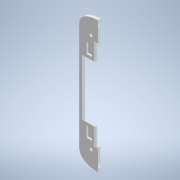
# Autodesk Inventor part: back_diffuser
Saved by Autodesk Inventor 2022 (Build 260153000, 153)
## iProperties
Created: 2024-12-22
Part Number: back_diffuser
Material: Типовые
Document SubType Name: Modeling
Designer: Andrey
Density: 1 g/cm^3
Appearance: По умолчанию
Author: Andrey
Autodesk Inventor part; units mm, degrees
ref_plane "YZ Plane" through (0, 0, 0) normal (1, 0, 0) x (0, 1, 0)
ref_plane "XZ Plane" through (0, 0, 0) normal (0, 1, 0) x (-1, 0, 0)
ref_plane "XY Plane" through (0, 0, 0) normal (0, 0, 1) x (1, 0, 0)
sketch "Эскиз1" plane through (0, 0, 0) normal (0, 0, 1) x (1, 0, 0)
  arc A0 (21.9698, 25.0872) -> (24.9698, 22.0872) centre (24.9698, 25.0872) ccw
  line L0 (24.9698, 22.0872) -> (32.4715, 22.0872)
  arc A1 (35.4715, 19.0872) -> (32.4715, 22.0872) centre (32.4715, 19.0872) ccw
  line L1 (35.4715, 19.0872) -> (35.4715, -12.1128)
  arc A2 (32.4715, -15.1128) -> (35.4715, -12.1128) centre (32.4715, -12.1128) ccw
  line L2 (32.4715, -15.1128) -> (24.9698, -15.1128)
  arc A3 (24.9698, -15.1128) -> (21.9698, -18.1128) centre (24.9698, -18.1128) ccw
  line L3 (21.9698, -18.1128) -> (21.9698, -28.1128)
  line L4 (21.9698, -28.1128) -> (36.9698, -28.1128)
  line L5 (36.9698, -28.1128) -> (36.9698, -40.6128)
  line L6 (36.9698, -40.6128) -> (21.9698, -40.6128)
  line L7 (21.9698, -40.6128) -> (21.9698, -43.5128)
  line L8 (21.9698, -43.5128) -> (58.0248, -43.5128)
  arc A4 (60.0248, -45.5128) -> (58.0248, -43.5128) centre (58.0248, -45.5128) ccw
  line L9 (60.0248, -45.5128) -> (60.0248, -60.8075)
  arc A5 (58.0248, -62.8075) -> (60.0248, -60.8075) centre (58.0248, -60.8075) ccw
  line L10 (58.0248, -62.8075) -> (-57.9752, -62.8075)
  arc A6 (-59.9752, -60.8075) -> (-57.9752, -62.8075) centre (-57.9752, -60.8075) ccw
  line L11 (-59.9752, -60.8075) -> (-59.9752, -45.5128)
  arc A7 (-57.9752, -43.5128) -> (-59.9752, -45.5128) centre (-57.9752, -45.5128) ccw
  line L12 (-57.9752, -43.5128) -> (-22.0457, -43.5128)
  line L13 (-22.0457, -43.5128) -> (-22.0457, -40.6128)
  line L14 (-22.0457, -40.6128) -> (-39.5957, -40.6128)
  line L15 (-39.5957, -40.6128) -> (-39.5957, -29.6128)
  line L16 (-39.5957, -29.6128) -> (-22.0457, -29.6128)
  line L17 (-22.0457, -29.6128) -> (-22.0457, -27.6266)
  line L18 (-22.0457, -27.6266) -> (-23.1715, -27.6266)
  line L19 (-23.1715, -27.6266) -> (-23.1715, -10.2508)
  line L20 (-23.1715, -10.2508) -> (-22.0457, -10.2508)
  line L21 (-22.0457, -10.2508) -> (-22.0457, -5.0128)
  line L22 (-22.0457, -5.0128) -> (-25.0457, -5.0128)
  line L23 (-25.0457, -5.0128) -> (-25.0457, 4.9872)
  line L24 (-25.0457, 4.9872) -> (-22.0457, 4.9872)
  line L25 (-22.0457, 4.9872) -> (-22.0457, 10.2252)
  line L26 (-22.0457, 10.2252) -> (-23.1715, 10.2252)
  line L27 (-23.1715, 10.2252) -> (-23.1715, 27.601)
  line L28 (-23.1715, 27.601) -> (-22.0457, 27.601)
  line L29 (-22.0457, 27.601) -> (-22.0457, 43.4872)
  line L30 (-22.0457, 43.4872) -> (-57.9752, 43.4872)
  arc A8 (-59.9752, 45.4872) -> (-57.9752, 43.4872) centre (-57.9752, 45.4872) ccw
  line L31 (-59.9752, 45.4872) -> (-59.9752, 60.782)
  arc A9 (-57.9752, 62.782) -> (-59.9752, 60.782) centre (-57.9752, 60.782) ccw
  line L32 (-57.9752, 62.782) -> (58.0248, 62.782)
  arc A10 (60.0248, 60.782) -> (58.0248, 62.782) centre (58.0248, 60.782) ccw
  line L33 (60.0248, 60.782) -> (60.0248, 45.4872)
  arc A11 (58.0248, 43.4872) -> (60.0248, 45.4872) centre (58.0248, 45.4872) ccw
  line L34 (58.0248, 43.4872) -> (21.9698, 43.4872)
  line L35 (21.9698, 43.4872) -> (21.9698, 25.0872)
  circle A12 centre (-51.6466, 22.9919) radius 1.5
  circle A13 centre (-51.6466, -23.0174) radius 1.5
  line L36 (-50.445, -3.8128) -> (-50.445, 15.6872)
  arc A14 (-47.445, 18.6872) -> (-50.445, 15.6872) centre (-47.445, 15.6872) ccw
  line L37 (-47.445, 18.6872) -> (-33.6813, 18.6872)
  arc A15 (-30.6813, 15.6872) -> (-33.6813, 18.6872) centre (-33.6813, 15.6872) ccw
  line L38 (-30.6813, 15.6872) -> (-30.6813, -3.8128)
  arc A16 (-33.6813, -6.8128) -> (-30.6813, -3.8128) centre (-33.6813, -3.8128) ccw
  line L39 (-33.6813, -6.8128) -> (-47.445, -6.8128)
  arc A17 (-50.445, -3.8128) -> (-47.445, -6.8128) centre (-47.445, -3.8128) ccw
  line L40 (60.4248, -29.3128) -> (60.4248, -21.9128)
  line L41 (60.4248, -21.9128) -> (74.9248, -21.9128)
  line L42 (74.9248, -21.9128) -> (74.9248, -29.3128)
  line L43 (74.9248, -29.3128) -> (60.4248, -29.3128)
  line L44 (60.4248, 21.8872) -> (60.4248, 29.2872)
  line L45 (60.4248, 29.2872) -> (74.9248, 29.2872)
  line L46 (74.9248, 29.2872) -> (74.9248, 21.8872)
  line L47 (74.9248, 21.8872) -> (60.4248, 21.8872)
  line L48 (79.0248, -17.5128) -> (68.0248, -17.5128)
  line L49 (68.0248, -17.5128) -> (68.0248, -6.0128)
  line L50 (68.0248, -6.0128) -> (63.1715, -6.0128)
  arc A18 (62.1715, -5.0128) -> (63.1715, -6.0128) centre (63.1715, -5.0128) ccw
  line L51 (62.1715, -5.0128) -> (62.1715, 4.9872)
  arc A19 (63.1715, 5.9872) -> (62.1715, 4.9872) centre (63.1715, 4.9872) ccw
  line L52 (63.1715, 5.9872) -> (68.0248, 5.9872)
  line L53 (68.0248, 5.9872) -> (68.0248, 17.4872)
  line L54 (68.0248, 17.4872) -> (79.0248, 17.4872)
  line L55 (79.0248, 17.4872) -> (79.0248, 52.7508)
  spline S0 degree 4 poles (79.0248, 52.7508) (79.0248, 55.4389) (78.6593, 58.1507) (77.2994, 60.4709) (75.0248, 62.2967) knots 0 0 0 0 0 1 1 1 1 1
  spline S1 degree 4 poles (75.0248, 62.2967) (71.8239, 64.8662) (66.8118, 66.4567) (60.2111, 66.782) (55.0248, 66.782) knots 0.415412 0.415412 0.415412 0.415412 0.415412 1 1 1 1 1
  line L56 (-54.9752, 66.782) -> (55.0248, 66.782)
  spline S2 degree 4 poles (-54.9752, 66.782) (-60.1615, 66.782) (-66.7622, 66.4567) (-71.7743, 64.8662) (-74.9752, 62.2967) knots 0 0 0 0 0 0.584588 0.584588 0.584588 0.584588 0.584588
  spline S3 degree 4 poles (-74.9752, 62.2967) (-77.2498, 60.4709) (-78.6098, 58.1507) (-78.9752, 55.4389) (-78.9752, 52.7508) knots 0 0 0 0 0 1 1 1 1 1
  line L57 (-78.9752, 52.7508) -> (-78.9752, -52.7764)
  spline S4 degree 4 poles (-78.9752, -52.7764) (-78.9752, -55.4644) (-78.6098, -58.1763) (-77.2498, -60.4964) (-74.9752, -62.3223) knots 0 0 0 0 0 1 1 1 1 1
  spline S5 degree 4 poles (-74.9752, -62.3223) (-71.7743, -64.8917) (-66.7622, -66.4822) (-60.1615, -66.8075) (-54.9752, -66.8075) knots 0.415412 0.415412 0.415412 0.415412 0.415412 1 1 1 1 1
  line L58 (55.0248, -66.8075) -> (-54.9752, -66.8075)
  spline S6 degree 4 poles (55.0248, -66.8075) (60.2111, -66.8075) (66.8118, -66.4822) (71.8239, -64.8917) (75.0248, -62.3223) knots 0 0 0 0 0 0.584588 0.584588 0.584588 0.584588 0.584588
  spline S7 degree 4 poles (75.0248, -62.3223) (77.2994, -60.4964) (78.6593, -58.1763) (79.0248, -55.4644) (79.0248, -52.7764) knots 0 0 0 0 0 1 1 1 1 1
  line L59 (79.0248, -52.7764) -> (79.0248, -17.5128)
  circle A20 centre (-29.4752, -25.5128) radius 1.25
  circle A21 centre (29.5248, 25.4872) radius 1.25
  circle A22 centre (29.5248, -25.5128) radius 1.25
  circle A23 centre (-29.4752, 25.4872) radius 1.25
  circle A24 centre (-51.6466, 22.9919) radius 2.1
  circle A25 centre (-51.6466, -23.0174) radius 2.1
  line L60 (-72.9752, -28.1266) -> (-39.8957, -28.1266)
  line L61 (-39.8957, 28.101) -> (-72.9752, 28.101)
  line L62 (-39.8957, 28.101) -> (-39.8957, 16.9648)
  ellipse E0 centre (-48.5541, 13.1872) end of major axis (-34.5198, 13.1872) minor radius 4.8 (-39.8957, 16.9648) -> (-62.5883, 13.1872) ccw
  line L63 (-62.5883, 13.1872) -> (-62.5883, -1.3128)
  ellipse E1 centre (-48.5541, -1.3128) end of major axis (-62.5883, -1.3128) minor radius 4.8 (-62.5883, -1.3128) -> (-39.8957, -5.0904) ccw
  line L64 (-39.8957, -5.0904) -> (-39.8957, -28.1266)
  line L65 (-59.9752, -66.667) -> (-59.9752, 66.6415)
  line L66 (-75.9752, -52.7764) -> (-75.9752, 52.7508)
  line L67 (-54.9752, 63.782) -> (55.0248, 63.782)
  line L68 (76.0248, 52.7508) -> (76.0248, 20.4872)
  line L69 (76.0248, 20.4872) -> (65.0248, 20.4872)
  line L70 (65.0248, 20.4872) -> (65.0248, 8.9872)
  line L71 (65.0248, 8.9872) -> (63.1715, 8.9872)
  arc A26 (63.1715, 8.9872) -> (59.1715, 4.9872) centre (63.1715, 4.9872) ccw
  line L72 (59.1715, 4.9872) -> (59.1715, -5.0128)
  arc A27 (59.1715, -5.0128) -> (63.1715, -9.0128) centre (63.1715, -5.0128) ccw
  line L73 (63.1715, -9.0128) -> (65.0248, -9.0128)
  line L74 (65.0248, -9.0128) -> (65.0248, -20.5128)
  line L75 (65.0248, -20.5128) -> (76.0248, -20.5128)
  line L76 (76.0248, -20.5128) -> (76.0248, -52.7764)
  line L77 (55.0248, -63.8075) -> (-54.9752, -63.8075)
  line L78 (-72.9752, -28.1266) -> (-72.9752, 28.101)
  spline S8 degree 5 poles (-73.0972, -59.9828) (-73.6957, -59.5017) (-74.2433, -58.9582) (-74.7152, -58.3353) (-75.4815, -56.9001) (-75.8411, -55.3112) (-75.9357, -54.4671) (-75.9756, -53.6221) (-75.9752, -52.7764) knots 0 0 0 0 0 0 0.475904 0.475904 0.475904 1 1 1 1 1 1
  spline S9 degree 5 poles (-75.9752, 52.7508) (-75.9756, 53.5966) (-75.9357, 54.4415) (-75.8411, 55.2856) (-75.4815, 56.8745) (-74.7152, 58.3097) (-74.2433, 58.9326) (-73.6957, 59.4761) (-73.0972, 59.9572) knots 0 0 0 0 0 0 0.524096 0.524096 0.524096 1 1 1 1 1 1
  spline S10 degree 5 poles (-73.0972, 59.9572) (-71.8214, 60.9817) (-70.3144, 61.7034) (-68.7678, 62.2382) (-65.1123, 63.1767) (-61.3615, 63.5924) (-59.2342, 63.7293) (-57.1048, 63.7818) (-54.9752, 63.782) knots 0 0 0 0 0 0 0.434284 0.434284 0.434284 1 1 1 1 1 1
  spline S11 degree 5 poles (55.0248, 63.782) (57.1544, 63.7818) (59.2838, 63.7293) (61.4111, 63.5924) (65.1619, 63.1767) (68.8174, 62.2382) (70.364, 61.7034) (71.871, 60.9817) (73.1468, 59.9572) knots 0 0 0 0 0 0 0.565716 0.565716 0.565716 1 1 1 1 1 1
  spline S12 degree 5 poles (73.1468, 59.9572) (73.7453, 59.4761) (74.2929, 58.9326) (74.7647, 58.3097) (75.531, 56.8745) (75.8907, 55.2856) (75.9853, 54.4415) (76.0252, 53.5966) (76.0248, 52.7508) knots 0 0 0 0 0 0 0.475904 0.475904 0.475904 1 1 1 1 1 1
  spline S13 degree 5 poles (76.0248, -52.7764) (76.0252, -53.6221) (75.9853, -54.4671) (75.8907, -55.3112) (75.531, -56.9001) (74.7647, -58.3353) (74.2929, -58.9582) (73.7453, -59.5017) (73.1468, -59.9828) knots 0 0 0 0 0 0 0.524096 0.524096 0.524096 1 1 1 1 1 1
  spline S14 degree 5 poles (73.1468, -59.9828) (71.871, -61.0073) (70.364, -61.7289) (68.8174, -62.2638) (65.1619, -63.2022) (61.4111, -63.618) (59.2838, -63.7549) (57.1544, -63.8074) (55.0248, -63.8075) knots 0 0 0 0 0 0 0.434284 0.434284 0.434284 1 1 1 1 1 1
  spline S15 degree 5 poles (-54.9752, -63.8075) (-57.1048, -63.8074) (-59.2342, -63.7549) (-61.3615, -63.618) (-65.1123, -63.2022) (-68.7678, -62.2638) (-70.3144, -61.7289) (-71.8214, -61.0073) (-73.0972, -59.9828) knots 0 0 0 0 0 0 0.565716 0.565716 0.565716 1 1 1 1 1 1
  point P0 (0, 0)
  point P1 (-78.9752, -28.1266)
  point P2 (-78.9752, 28.101)
  point P3 (-59.9752, -63.6611)
  point P4 (-59.9752, 63.6356)
  dimension "d0" = 3
  constraints: 26 end point, 8 parallel, 4 point on circle, 2 centre point, 1 collinear, 38 other
extrude "Выдавливание1" add sketch "Эскиз1" along normal blind 3 contours S10 S9 L66 S8 S15 L65 S5 S4 L57 S3 S2
sketch "Эскиз3" plane through (0, 0, 3) normal (0, 0, 1) x (1, 0, 0)
  line L0 (-78.9752, 52.7508) -> (-78.9752, -52.7764) projected
  line L1 (-59.9752, -66.667) -> (-59.9752, -63.6611) projected
  spline S0 degree 5 poles (-59.9752, -63.6611) (-61.1018, -63.5885) (-62.2267, -63.4897) (-63.3488, -63.36) (-66.084, -62.9528) (-68.7678, -62.2638) (-70.3144, -61.7289) (-71.8214, -61.0073) (-73.0972, -59.9828) knots 0 0 0 0 0 0 0.408481 0.408481 0.408481 1 1 1 1 1 1 projected
  spline S1 degree 5 poles (-73.0972, -59.9828) (-73.6957, -59.5017) (-74.2433, -58.9582) (-74.7152, -58.3353) (-75.4815, -56.9001) (-75.8411, -55.3112) (-75.9357, -54.4671) (-75.9756, -53.6221) (-75.9752, -52.7764) knots 0 0 0 0 0 0 0.475904 0.475904 0.475904 1 1 1 1 1 1 projected
  line L2 (-75.9752, -52.7764) -> (-75.9752, 52.7508) projected
  spline S2 degree 5 poles (-75.9752, 52.7508) (-75.9756, 53.5966) (-75.9357, 54.4415) (-75.8411, 55.2856) (-75.4815, 56.8745) (-74.7152, 58.3097) (-74.2433, 58.9326) (-73.6957, 59.4761) (-73.0972, 59.9572) knots 0 0 0 0 0 0 0.524096 0.524096 0.524096 1 1 1 1 1 1 projected
  spline S3 degree 5 poles (-73.0972, 59.9572) (-71.8214, 60.9817) (-70.3144, 61.7034) (-68.7678, 62.2382) (-66.084, 62.9272) (-63.3488, 63.3345) (-62.2267, 63.4641) (-61.1018, 63.5629) (-59.9752, 63.6355) knots 0 0 0 0 0 0 0.591519 0.591519 0.591519 1 1 1 1 1 1 projected
  line L3 (-59.9752, 63.6356) -> (-59.9752, 66.6415) projected
  line L4 (-39.8957, 28.101) -> (-59.6752, 28.101) projected
  line L5 (-39.8957, 28.101) -> (-39.8957, 16.9648) projected
  circle A0 centre (-51.6466, 22.9919) radius 2.1 projected
  line L6 (-78.9752, -28.1266) -> (-76.3894, -28.1266) projected
  line L7 (-78.9752, 28.101) -> (-78.9752, -28.1266) projected
  line L8 (-76.3894, 28.101) -> (-78.9752, 28.101) projected
  line L9 (-59.9752, -66.667) -> (-59.9752, -63.6611) projected
  line L10 (-59.9752, -63.6611) -> (-59.9752, 63.6356)
  line L11 (-59.9752, -28.4266) -> (-78.9752, -28.4266)
  line L12 (-59.9752, 28.401) -> (-78.9752, 28.401)
  line L13 (-76.3894, -28.1266) -> (-76.3894, 28.101) projected
  ellipse E0 centre (-48.5541, 13.1872) end of major axis (-34.5198, 13.1872) minor radius 4.8 (-39.8957, 16.9648) -> (-59.6752, 16.115) ccw projected
  line L14 (-59.6752, 16.115) -> (-59.6752, 28.101) projected
  point P0 (0, 0)
  point P1 (-75.9752, 28.401)
  point P2 (-75.9752, -28.4266)
  dimension "d5" = 0.3
  constraints: 6 end point, 4 point on line, 2 perpendicular, 1 collinear, 9 other
  measures "d5" distance between parallel lines of L12 L4
extrude "Выдавливание3" add sketch "Эскиз3" against normal blind 0.4 contours L2 S2 S3 L10 L12 | L11 L10 S0 S1 L2
sketch "Эскиз4" plane through (0, 0, 2.6) normal (0, 0, -1) x (-1, 0, 0)
  circle A0 centre (66.9752, -50.0128) radius 1.35
  circle A1 centre (66.9752, 49.9872) radius 1.35
  arc A2 (57.945, -33.5297) -> (52.945, -33.5297) centre (55.445, -33.5297) ccw
  line L0 (57.945, -33.5297) -> (57.945, -38.6097)
  arc A3 (52.945, -38.6097) -> (57.945, -38.6097) centre (55.445, -38.6097) ccw
  line L1 (52.945, -38.6097) -> (52.945, -33.5297)
  line L2 (44.445, -39.1128) -> (44.445, -31.1128)
  arc A4 (45.445, -30.1128) -> (44.445, -31.1128) centre (45.445, -31.1128) ccw
  line L3 (45.445, -30.1128) -> (48.445, -30.1128)
  arc A5 (49.445, -31.1128) -> (48.445, -30.1128) centre (48.445, -31.1128) ccw
  line L4 (49.445, -31.1128) -> (49.445, -39.1128)
  arc A6 (48.445, -40.1128) -> (49.445, -39.1128) centre (48.445, -39.1128) ccw
  line L5 (48.445, -40.1128) -> (45.445, -40.1128)
  arc A7 (44.445, -39.1128) -> (45.445, -40.1128) centre (45.445, -39.1128) ccw
  arc A8 (40.445, -8.8128) -> (38.445, -6.8128) centre (38.445, -8.8128) ccw
  line L6 (38.445, -6.8128) -> (33.6813, -6.8128)
  arc A9 (30.6813, -3.8128) -> (33.6813, -6.8128) centre (33.6813, -3.8128) ccw
  line L7 (30.6813, -3.8128) -> (30.6813, 15.6872)
  arc A10 (33.6813, 18.6872) -> (30.6813, 15.6872) centre (33.6813, 15.6872) ccw
  line L8 (33.6813, 18.6872) -> (47.445, 18.6872)
  arc A11 (50.445, 15.6872) -> (47.445, 18.6872) centre (47.445, 15.6872) ccw
  line L9 (50.445, 15.6872) -> (50.445, -14.8128)
  arc A12 (48.445, -16.8128) -> (50.445, -14.8128) centre (48.445, -14.8128) ccw
  line L10 (48.445, -16.8128) -> (42.445, -16.8128)
  arc A13 (40.445, -14.8128) -> (42.445, -16.8128) centre (42.445, -14.8128) ccw
  line L11 (40.445, -14.8128) -> (40.445, -8.8128)
  circle A14 centre (51.6466, 22.9919) radius 1.5
  circle A15 centre (51.6466, -23.0174) radius 1.5
  line L12 (-60.4248, -21.9128) -> (-60.4248, -29.3128)
  line L13 (-60.4248, -29.3128) -> (-74.9248, -29.3128)
  line L14 (-74.9248, -29.3128) -> (-74.9248, -21.9128)
  line L15 (-74.9248, -21.9128) -> (-60.4248, -21.9128)
  line L16 (-60.4248, 29.2872) -> (-60.4248, 21.8872)
  line L17 (-60.4248, 21.8872) -> (-74.9248, 21.8872)
  line L18 (-74.9248, 21.8872) -> (-74.9248, 29.2872)
  line L19 (-74.9248, 29.2872) -> (-60.4248, 29.2872)
  line L20 (-68.0248, -17.5128) -> (-79.0248, -17.5128)
  line L21 (-79.0248, -52.7764) -> (-79.0248, -17.5128)
  spline S0 degree 4 poles (-75.0248, -62.3223) (-77.2994, -60.4964) (-78.6593, -58.1763) (-79.0248, -55.4644) (-79.0248, -52.7764) knots 0 0 0 0 0 1 1 1 1 1
  spline S1 degree 4 poles (-55.0248, -66.8075) (-60.2111, -66.8075) (-66.8118, -66.4822) (-71.8239, -64.8917) (-75.0248, -62.3223) knots 0 0 0 0 0 0.584588 0.584588 0.584588 0.584588 0.584588
  line L22 (54.9752, -66.8075) -> (-55.0248, -66.8075)
  spline S2 degree 4 poles (74.9752, -62.3223) (71.7743, -64.8917) (66.7622, -66.4822) (60.1615, -66.8075) (54.9752, -66.8075) knots 0.415412 0.415412 0.415412 0.415412 0.415412 1 1 1 1 1
  spline S3 degree 4 poles (78.9752, -52.7764) (78.9752, -55.4644) (78.6098, -58.1763) (77.2498, -60.4964) (74.9752, -62.3223) knots 0 0 0 0 0 1 1 1 1 1
  line L23 (78.9752, 52.7508) -> (78.9752, -52.7764)
  spline S4 degree 4 poles (74.9752, 62.2967) (77.2498, 60.4709) (78.6098, 58.1507) (78.9752, 55.4389) (78.9752, 52.7508) knots 0 0 0 0 0 1 1 1 1 1
  spline S5 degree 4 poles (54.9752, 66.782) (60.1615, 66.782) (66.7622, 66.4567) (71.7743, 64.8662) (74.9752, 62.2967) knots 0 0 0 0 0 0.584588 0.584588 0.584588 0.584588 0.584588
  line L24 (-55.0248, 66.782) -> (54.9752, 66.782)
  spline S6 degree 4 poles (-75.0248, 62.2967) (-71.8239, 64.8662) (-66.8118, 66.4567) (-60.2111, 66.782) (-55.0248, 66.782) knots 0.415412 0.415412 0.415412 0.415412 0.415412 1 1 1 1 1
  spline S7 degree 4 poles (-79.0248, 52.7508) (-79.0248, 55.4389) (-78.6593, 58.1507) (-77.2994, 60.4709) (-75.0248, 62.2967) knots 0 0 0 0 0 1 1 1 1 1
  line L25 (-79.0248, 17.4872) -> (-79.0248, 52.7508)
  line L26 (-79.0248, 17.4872) -> (-68.0248, 17.4872)
  line L27 (-68.0248, 17.4872) -> (-68.0248, 5.9872)
  line L28 (-68.0248, 5.9872) -> (-63.1715, 5.9872)
  arc A16 (-62.1715, 4.9872) -> (-63.1715, 5.9872) centre (-63.1715, 4.9872) ccw
  line L29 (-62.1715, 4.9872) -> (-62.1715, -5.0128)
  arc A17 (-63.1715, -6.0128) -> (-62.1715, -5.0128) centre (-63.1715, -5.0128) ccw
  line L30 (-63.1715, -6.0128) -> (-68.0248, -6.0128)
  line L31 (-68.0248, -6.0128) -> (-68.0248, -17.5128)
  circle A18 centre (29.4752, -25.5128) radius 1.25
  circle A19 centre (-29.5248, 25.4872) radius 1.25
  circle A20 centre (-29.5248, -25.5128) radius 1.25
  circle A21 centre (29.4752, 25.4872) radius 1.25
  arc A22 (-24.9698, 22.0872) -> (-21.9698, 25.0872) centre (-24.9698, 25.0872) ccw
  line L32 (-21.9698, 25.0872) -> (-21.9698, 43.4872)
  line L33 (-58.0248, 43.4872) -> (-21.9698, 43.4872)
  arc A23 (-60.0248, 45.4872) -> (-58.0248, 43.4872) centre (-58.0248, 45.4872) ccw
  line L34 (-60.0248, 45.4872) -> (-60.0248, 60.782)
  arc A24 (-58.0248, 62.782) -> (-60.0248, 60.782) centre (-58.0248, 60.782) ccw
  line L35 (-58.0248, 62.782) -> (57.9752, 62.782)
  arc A25 (59.9752, 60.782) -> (57.9752, 62.782) centre (57.9752, 60.782) ccw
  line L36 (59.9752, 60.782) -> (59.9752, 45.4872)
  arc A26 (57.9752, 43.4872) -> (59.9752, 45.4872) centre (57.9752, 45.4872) ccw
  line L37 (22.0457, 43.4872) -> (57.9752, 43.4872)
  line L38 (22.0457, 43.4872) -> (22.0457, 27.601)
  line L39 (22.0457, 27.601) -> (23.1715, 27.601)
  line L40 (23.1715, 27.601) -> (23.1715, 10.2252)
  line L41 (23.1715, 10.2252) -> (22.0457, 10.2252)
  line L42 (22.0457, 10.2252) -> (22.0457, 4.9872)
  line L43 (22.0457, 4.9872) -> (25.0457, 4.9872)
  line L44 (25.0457, 4.9872) -> (25.0457, -5.0128)
  line L45 (25.0457, -5.0128) -> (22.0457, -5.0128)
  line L46 (22.0457, -5.0128) -> (22.0457, -10.2508)
  line L47 (22.0457, -10.2508) -> (23.1715, -10.2508)
  line L48 (23.1715, -10.2508) -> (23.1715, -27.6266)
  line L49 (23.1715, -27.6266) -> (22.0457, -27.6266)
  line L50 (22.0457, -27.6266) -> (22.0457, -29.6128)
  line L51 (22.0457, -29.6128) -> (39.5957, -29.6128)
  line L52 (39.5957, -29.6128) -> (39.5957, -40.6128)
  line L53 (39.5957, -40.6128) -> (22.0457, -40.6128)
  line L54 (22.0457, -40.6128) -> (22.0457, -43.5128)
  line L55 (57.9752, -43.5128) -> (22.0457, -43.5128)
  arc A27 (59.9752, -45.5128) -> (57.9752, -43.5128) centre (57.9752, -45.5128) ccw
  line L56 (59.9752, -45.5128) -> (59.9752, -60.8075)
  arc A28 (57.9752, -62.8075) -> (59.9752, -60.8075) centre (57.9752, -60.8075) ccw
  line L57 (57.9752, -62.8075) -> (-58.0248, -62.8075)
  arc A29 (-60.0248, -60.8075) -> (-58.0248, -62.8075) centre (-58.0248, -60.8075) ccw
  line L58 (-60.0248, -60.8075) -> (-60.0248, -45.5128)
  arc A30 (-58.0248, -43.5128) -> (-60.0248, -45.5128) centre (-58.0248, -45.5128) ccw
  line L59 (-21.9698, -43.5128) -> (-58.0248, -43.5128)
  line L60 (-21.9698, -43.5128) -> (-21.9698, -40.6128)
  line L61 (-21.9698, -40.6128) -> (-36.9698, -40.6128)
  line L62 (-36.9698, -40.6128) -> (-36.9698, -28.1128)
  line L63 (-36.9698, -28.1128) -> (-21.9698, -28.1128)
  line L64 (-21.9698, -28.1128) -> (-21.9698, -18.1128)
  arc A31 (-21.9698, -18.1128) -> (-24.9698, -15.1128) centre (-24.9698, -18.1128) ccw
  line L65 (-24.9698, -15.1128) -> (-32.4715, -15.1128)
  arc A32 (-35.4715, -12.1128) -> (-32.4715, -15.1128) centre (-32.4715, -12.1128) ccw
  line L66 (-35.4715, -12.1128) -> (-35.4715, 19.0872)
  arc A33 (-32.4715, 22.0872) -> (-35.4715, 19.0872) centre (-32.4715, 19.0872) ccw
  line L67 (-32.4715, 22.0872) -> (-24.9698, 22.0872)
  circle A34 centre (66.9752, 49.9872) radius 1.6
  circle A35 centre (66.9752, -50.0128) radius 1.6
  point P0 (0, 0)
  dimension "d9" = 3.2
  dimension "d10" = 3.2
  constraints: 2 centre point, 2 coincident
  measures "d9" diameter of A34
  measures "d10" diameter of A35
extrude "Выдавливание4" cut sketch "Эскиз4" against normal blind 1 contours A0 | A1 | A34 | A35
sketch "Эскиз5" plane through (0, 0, 2.6) normal (0, 0, -1) x (-1, 0, 0)
  circle A0 centre (66.9752, 49.9872) radius 1.6
  circle A1 centre (66.9752, -50.0128) radius 1.6
  line L0 (78.9752, 52.7508) -> (78.9752, -52.7764)
  line L1 (59.9752, -66.667) -> (59.9752, -28.4266)
  line L2 (59.9752, -28.4266) -> (75.9752, -28.4266)
  line L3 (75.9752, -28.4266) -> (75.9752, 28.401)
  line L4 (75.9752, 28.401) -> (59.9752, 28.401)
  line L5 (59.9752, 28.401) -> (59.9752, 66.6415)
  line L6 (78.9752, 52.7508) -> (78.9752, -52.7764)
  spline S0 degree 4 poles (74.9752, 62.2967) (77.2498, 60.4709) (78.6098, 58.1507) (78.9752, 55.4389) (78.9752, 52.7508) knots 0 0 0 0 0 1 1 1 1 1
  spline S1 degree 4 poles (59.9752, 66.6415) (64.3981, 66.3697) (68.939, 65.6863) (72.4991, 64.2844) (74.9752, 62.2967) knots 0 0 0 0 0 1 1 1 1 1
  spline S2 degree 3 poles (73.0972, 59.9572) (72.8317, 60.1704) (72.2504, 60.5866) (71.3901, 61.0754) (70.4297, 61.5347) (69.5826, 61.8759) (68.4322, 62.2648) (67.4425, 62.5442) (66.1307, 62.8516) (65.027, 63.0635) (63.595, 63.2862) (62.4143, 63.4312) (61.1039, 63.5554) (60.3883, 63.6089) (59.9752, 63.6356) knots 0 0 0 0 0.108911 0.217823 0.272278 0.38119 0.435645 0.544557 0.599012 0.707924 0.762379 0.871291 0.925747 1 1 1 1
  spline S3 degree 3 poles (75.9752, 52.7508) (75.9752, 53.2802) (75.9431, 54.1752) (75.8223, 55.1158) (75.6926, 55.7827) (75.5863, 56.208) (75.4279, 56.7161) (75.2804, 57.1045) (75.0687, 57.5698) (74.8765, 57.9272) (74.6051, 58.3588) (74.3614, 58.6932) (74.0195, 59.1004) (73.638, 59.4977) (73.2859, 59.8058) (73.0972, 59.9572) knots 0 0 0 0 0.166667 0.291667 0.333333 0.416667 0.458333 0.541667 0.583333 0.666667 0.708333 0.791667 0.833333 0.916667 1 1 1 1
  line L7 (75.9752, -52.7764) -> (75.9752, 52.7508)
  spline S4 degree 3 poles (73.0972, -59.9828) (73.2859, -59.8313) (73.638, -59.5233) (74.0195, -59.126) (74.3614, -58.7188) (74.6051, -58.3843) (74.8765, -57.9527) (75.0687, -57.5953) (75.2804, -57.1301) (75.4279, -56.7417) (75.5863, -56.2336) (75.6926, -55.8083) (75.8007, -55.2525) (75.8676, -54.7887) (75.9281, -54.186) (75.9662, -53.5615) (75.9752, -53.0411) (75.9752, -52.7764) knots 0 0 0 0 0.083333 0.166667 0.208333 0.291667 0.333333 0.416667 0.458333 0.541667 0.583333 0.666667 0.708333 0.791667 0.833333 0.916667 1 1 1 1
  spline S5 degree 3 poles (59.9752, -63.6611) (60.3883, -63.6345) (61.1039, -63.581) (62.4143, -63.4568) (63.595, -63.3118) (65.027, -63.0891) (66.1307, -62.8772) (67.4425, -62.5698) (68.4322, -62.2903) (69.5826, -61.9014) (70.4297, -61.5602) (71.3901, -61.101) (72.2504, -60.6122) (72.8317, -60.196) (73.0972, -59.9828) knots 0 0 0 0 0.074253 0.128709 0.237621 0.292076 0.400988 0.455443 0.564355 0.61881 0.727722 0.782177 0.891089 1 1 1 1
  spline S6 degree 4 poles (74.9752, -62.3223) (72.4991, -64.31) (68.939, -65.7118) (64.3981, -66.3953) (59.9752, -66.667) knots 0 0 0 0 0 1 1 1 1 1
  spline S7 degree 4 poles (78.9752, -52.7764) (78.9752, -55.4644) (78.6098, -58.1763) (77.2498, -60.4964) (74.9752, -62.3223) knots 0 0 0 0 0 1 1 1 1 1
  line L8 (71.9752, 52.7508) -> (71.9752, -52.7764)
  spline S8 degree 5 poles (59.7179, 59.6438) (61.136, 59.5524) (62.551, 59.417) (63.9606, 59.2241) (66.2021, 58.8052) (68.3651, 58.0878) (69.1524, 57.7616) (69.9266, 57.3714) (70.5933, 56.8379) knots 0 0 0 0 0 0 0.624879 0.624879 0.624879 1 1 1 1 1 1
  spline S9 degree 5 poles (70.5933, 56.8379) (70.8602, 56.6226) (71.1092, 56.3872) (71.3311, 56.1151) (71.7518, 55.3124) (71.9043, 54.4128) (71.9552, 53.862) (71.9752, 53.3056) (71.9752, 52.7508) knots 0 0 0 0 0 0 0.381774 0.381774 0.381774 1 1 1 1 1 1
  spline S10 degree 5 poles (71.9752, -52.7764) (71.9754, -53.3312) (71.9552, -53.8876) (71.9042, -54.4384) (71.7518, -55.338) (71.3311, -56.1407) (71.1092, -56.4128) (70.8602, -56.6482) (70.5933, -56.8635) knots 0 0 0 0 0 0 0.618226 0.618226 0.618226 1 1 1 1 1 1
  spline S11 degree 5 poles (70.5933, -56.8635) (69.9266, -57.397) (69.1524, -57.7871) (68.3651, -58.1134) (66.2021, -58.8308) (63.9606, -59.2497) (62.551, -59.4425) (61.136, -59.578) (59.7179, -59.6694) knots 0 0 0 0 0 0 0.375121 0.375121 0.375121 1 1 1 1 1 1
  point P0 (0, 0)
  point P1 (71.9752, -28.4266)
  point P2 (59.9752, -59.6522)
  point P3 (59.9752, 59.6267)
  point P4 (71.9752, 28.401)
  dimension "d20" = 4
  constraints: 2 end point, 2 parallel, 36 other
extrude "Выдавливание5" add sketch "Эскиз5" along normal blind 1.9 contours S8 S9 L8 L4 L5 | L1 L2 L8 S10 S11
sketch "Эскиз7" plane through (0, 0, 3) normal (0, 0, 1) x (1, 0, 0)
  circle A0 centre (-66.9752, 49.9872) radius 1.6 projected
  circle A1 centre (-66.9752, -50.0128) radius 1.6 projected
  line L0 (-78.9752, 52.7508) -> (-78.9752, -52.7764) projected
  line L1 (-59.9752, -66.667) -> (-59.9752, -28.4266) projected
  line L2 (-59.9752, -28.4266) -> (-75.9752, -28.4266) projected
  line L3 (-75.9752, -28.4266) -> (-75.9752, 28.401) projected
  line L4 (-75.9752, 28.401) -> (-59.9752, 28.401) projected
  line L5 (-59.9752, 28.401) -> (-59.9752, 66.6415) projected
  line L6 (-71.2752, 31.701) -> (-66.2752, 31.701)
  line L7 (-66.2752, 31.701) -> (-66.2752, 41.701)
  line L8 (-66.2752, 41.701) -> (-71.2752, 41.701)
  line L9 (-71.2752, 41.701) -> (-71.2752, 31.701)
  line L10 (-71.2752, 31.701) -> (-66.2752, 41.701) construction
  line L11 (-66.2752, 31.701) -> (-71.2752, 41.701) construction
  line L12 (-65.9752, 42.001) -> (-65.9752, 31.401)
  line L13 (-65.9752, 31.401) -> (-71.5752, 31.401)
  line L14 (-71.5752, 31.401) -> (-71.5752, 42.001)
  line L15 (-71.5752, 42.001) -> (-65.9752, 42.001)
  point P0 (0, 0)
  point P1 (-68.7752, 36.701)
  dimension "d38" = 5
  dimension "d39" = 10
  dimension "d40" = 0.3
  dimension "d41" = 3
  dimension "d42" = 6
  constraints: 20 end point, 4 parallel, 2 midpoint, 2 perpendicular, 1 horizontal, 7 other
  measures "d38" distance of L8.end L7.end
  measures "d39" distance of L7.end L6.end
  measures "d40" distance between parallel lines of L7 L12
  measures "d41" distance between parallel lines of L13 L4
  measures "d42" distance between parallel lines of L5 L12
extrude "Выдавливание7" cut sketch "Эскиз7" against normal blind 1.8 contours L9 L8 L7 L6 | L12 L13 L14 L15
sketch "Эскиз8" plane through (0, 0, 3) normal (0, 0, 1) x (1, 0, 0)
  line L0 (-65.9752, 31.401) -> (-71.5752, 31.401) projected
  line L1 (-71.5752, 31.401) -> (-71.5752, 42.001) projected
  line L2 (-71.5752, 42.001) -> (-65.9752, 42.001) projected
  line L3 (-65.9752, 42.001) -> (-65.9752, 31.401) projected
  circle A0 centre (-66.9752, 49.9872) radius 1.6 projected
  circle A1 centre (-66.9752, -50.0128) radius 1.6 projected
  line L4 (-78.9752, 52.7508) -> (-78.9752, -52.7764) projected
  line L5 (-59.9752, -66.667) -> (-59.9752, -28.4266) projected
  line L6 (-59.9752, -28.4266) -> (-75.9752, -28.4266) projected
  line L7 (-75.9752, -28.4266) -> (-75.9752, 28.401) projected
  line L8 (-75.9752, 28.401) -> (-59.9752, 28.401) projected
  line L9 (-59.9752, 28.401) -> (-59.9752, 66.6415) projected
  line L10 (-61.6823, 45.001) -> (-72.9672, 45.001) projected
  line L11 (-59.9752, 28.401) -> (-71.9752, 28.401) projected
  line L12 (-59.9752, 28.401) -> (-62.9752, 28.401)
  line L13 (-62.9752, 28.401) -> (-62.9752, 45.001)
  line L14 (-62.9752, 45.001) -> (-59.9752, 45.001)
  line L15 (-59.9752, 45.001) -> (-59.9752, 28.401)
  line L16 (-59.9752, 28.401) -> (-59.9752, 66.6415) projected
  line L17 (-62.9752, 45.001) -> (-59.9752, 45.001)
  line L18 (-59.9752, 45.001) -> (-59.9752, 45.251)
  line L19 (-59.9752, 45.251) -> (-62.9752, 45.251)
  line L20 (-62.9752, 45.251) -> (-62.9752, 45.001)
  point P0 (0, 0)
  dimension "d45" = 3
  dimension "d48" = 0.25
  constraints: 16 end point, 4 parallel, 2 horizontal, 2 perpendicular, 2 point on line, 4 other
  measures "d45" distance of L13.end L14.end
  measures "d48" distance of L18.end L17.end
extrude "Выдавливание8" cut sketch "Эскиз8" against normal blind 3 contours L13 L10 L14 L9 L8 | L20 L19 L9 L14 L10
chamfer "Фаска3" distance 1 angle 45 2 edges at (-61.4752, 45.251, 3) (-62.9752, 36.826, 3)
mirror "Зеркальное отражение1" about plane through (0, 0, 0) normal (0, 1, 0) of "Выдавливание7", "Выдавливание8", "Фаска3"
